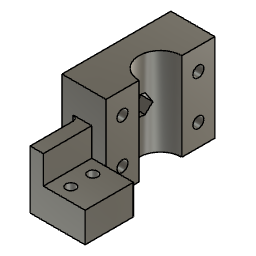
VI LC Clamp v1.0 (Autodesk Fusion 360 design; units mm, degrees)
Autodesk Fusion 360 part; units mm, degrees
note: some values were not read from the file. Set by a fixed rule: which sketch regions a step uses.
sketch "Sketch1" plane through (0, 0, 0) normal (0, 0, 1) x (1, 0, 0)
  circle A0 centre (0, 0) radius 9.75
  line L0 (0.0224, 9.75) -> (0.0224, 24.75)
  line L1 (0.0224, 24.75) -> (-19.9776, 24.75)
  line L2 (-19.9776, 24.75) -> (-19.9776, -24.75)
  line L3 (-19.9776, -24.75) -> (0, -24.75)
  line L4 (0, -24.75) -> (0, -9.75)
  line L5 (0, -24.75) -> (6.5, -24.75) construction
  line L6 (0, -24.75) -> (-6.5, -24.75) construction
  line L7 (-6.5, -24.75) -> (-6.5, -46.75)
  line L8 (-6.5, -46.75) -> (12.5, -46.75)
  line L9 (12.5, -46.75) -> (12.5, -25)
  line L10 (-6.5, -24.75) -> (-12.5, -24.75)
  line L11 (-12.5, -24.75) -> (-12.5, -46.75)
  line L12 (0, -24.75) -> (12.5, -24.75)
  line L13 (12.5, -24.75) -> (12.5, -25)
  line L14 (-6.5, -46.75) -> (-12.5, -46.75)
  dimension "d1" = 19.5
  dimension "d2" = 15
  dimension "d3" = 20
  dimension "d4" = 49.5
  dimension "d5" = 6.5
  dimension "d6" = 6.5
  dimension "d7" = 22
  dimension "d8" = 19
  dimension "d9" = 6
  constraint coincident A0.centre origin
  constraint coincident A0 L0.start
  constraint vertical L0
  constraint perpendicular L0 L1
  constraint perpendicular L1 L2
  constraint perpendicular L2 L3
  constraint coincident A0 L4.end
  constraint perpendicular L3 L4
  constraint perpendicular L4 L5
  constraint perpendicular L4 L6
  constraint perpendicular L3 L7
  constraint perpendicular L7 L8
  constraint perpendicular L8 L9
  constraint perpendicular L7 L10
  constraint perpendicular L3 L11
  constraint perpendicular L4 L12
  constraint perpendicular L11 L14
  measures "d1" diameter of A0
  measures "d2" distance of L0.start L0.end
  measures "d3" distance of L0.end L1.end
  measures "d4" distance of L1.end L2.end
  measures "d5" distance of L3.end L5.end
  measures "d6" distance of L3.end L6.end
  measures "d7" distance of L6.end L7.end
  measures "d8" distance of L7.end L8.end
  measures "d9" distance of L6.end L10.end
extrude "Extrude1" add sketch "Sketch1" along normal blind 40 contours A0 L0 L1 L2 L3 L4 L10
extrude "Extrude2" add sketch "Sketch1" along normal blind 13.6 contours L3 L7 L8 L9 L12 L13
extrude "Extrude3" add sketch "Sketch1" along normal blind 26.4 contours L3 L7 L10 L11 L14
sketch "Sketch2" plane through (-19.9776, 0, 0) normal (-1, 0, 0) x (0, -1, 0)
  line L0 (-24.75, 0) -> (24.75, 0)
  line L1 (24.75, 0) -> (24.75, 40)
  line L2 (24.75, 40) -> (-24.75, 40)
  line L3 (-24.75, 40) -> (-24.75, 0)
  line L4 (0, 40) -> (-9.75, 40) construction
  line L5 (-24.75, 40) -> (-17.25, 40) construction
  line L6 (-17.25, 40) -> (-17.25, 30) construction
  circle A0 centre (-17.25, 30) radius 2.5
  circle A1 centre (17.25, 30) radius 2.5
  circle A2 centre (-17.25, 10) radius 2.5
  circle A3 centre (17.25, 10) radius 2.5
  dimension "d16" = 9.75
  dimension "d17" = 7.5
  dimension "d18" = 10
  dimension "d20" = 5
  dimension "d23" = 34.5
  dimension "d24" = -20
  constraint midpoint L2 L4.start
  constraint perpendicular L1 L4
  constraint coincident L2.end L3.start
  constraint perpendicular L3 L5
  constraint perpendicular L0 L6
  constraint coincident L6.end A0.centre
  measures "d16" distance of L4.start L4.end
  measures "d17" distance of L2.end L5.end
  measures "d18" distance of L5.end L6.end
  measures "d20" diameter of A0
extrude "Extrude4" cut sketch "Sketch2" against normal blind 30 contours A0 | A1 | A2 | A3
sketch "Sketch3" plane through (0, 0, 13.6) normal (0, 0, 1) x (-1, 0, 0)
  line L0 (6.5, 24.75) -> (6.5, 46.75)
  line L1 (6.5, 46.75) -> (-12.5, 46.75)
  line L2 (-12.5, 46.75) -> (-12.5, 25)
  line L3 (0, 24.75) -> (6.5, 24.75)
  line L4 (-12.5, 25) -> (-12.5, 24.75)
  line L5 (-12.5, 24.75) -> (0, 24.75)
  line L6 (0, 24.75) -> (0, 30.75) construction
  circle A0 centre (0, 30.75) radius 2.25
  circle A1 centre (0, 40.75) radius 2.25
  dimension "d28" = 6
  dimension "d29" = 4.5
  dimension "d32" = 0
  dimension "d33" = 10
  constraint coincident L3.start L5.end
  constraint perpendicular L5 L6
  constraint coincident L6.end A0.centre
  measures "d28" distance of L3.start L6.end
  measures "d29" diameter of A0
extrude "Extrude5" cut sketch "Sketch3" against normal blind 14 contours A0 | A1
sketch "Sketch4" plane through (-19.9776, 0, 0) normal (-1, 0, 0) x (0, -1, 0)
  circle A0 centre (17.25, 30) radius 2.5
  circle A1 centre (17.25, 10) radius 2.5
  circle A2 centre (-17.25, 30) radius 2.5
  circle A3 centre (-17.25, 10) radius 2.5
  line L0 (-24.75, 0) -> (24.75, 0)
  line L1 (24.75, 0) -> (24.75, 40)
  line L2 (24.75, 40) -> (-24.75, 40)
  line L3 (-24.75, 40) -> (-24.75, 0)
  line L4 (0, 40) -> (0, 0) construction
  circle A4 centre (0, 20) radius 2.5
  dimension "d36" = 5
  constraint midpoint L2 L4.start
  constraint coincident L4.end origin
  constraint midpoint L4 A4.centre
  measures "d36" diameter of A4
extrude "Extrude6" cut sketch "Sketch4" against normal blind 20 contours A4
sketch "Sketch5" plane through (-19.9776, 0, 0) normal (-1, 0, 0) x (0, -1, 0)
  circle A0 centre (0, 20) radius 2.5
  circle A1 centre (17.25, 30) radius 2.5
  circle A2 centre (17.25, 10) radius 2.5
  circle A3 centre (-17.25, 30) radius 2.5
  circle A4 centre (-17.25, 10) radius 2.5
  line L0 (-24.75, 0) -> (24.75, 0)
  line L1 (24.75, 0) -> (24.75, 40)
  line L2 (24.75, 40) -> (-24.75, 40)
  line L3 (-24.75, 40) -> (-24.75, 0)
  line L4 (0, 20) -> (2.5, 24.3301) construction
  line L5 (0, 20) -> (5, 20) construction
  line L6 (0, 20) -> (-2.5, 24.3301) construction
  line L7 (0, 20) -> (5, 20) construction
  line L8 (0, 20) -> (-5, 20) construction
  line L9 (0, 20) -> (2.5, 15.6699) construction
  line L10 (-2.5, 15.6699) -> (0, 20) construction
  line L11 (5, 20) -> (2.5, 15.6699)
  line L12 (2.5, 15.6699) -> (-2.5, 15.6699)
  line L13 (-2.5, 15.6699) -> (-5, 20)
  line L14 (-5, 20) -> (-2.5, 24.3301)
  line L15 (-2.5, 24.3301) -> (2.5, 24.3301)
  line L16 (2.5, 24.3301) -> (5, 20)
  dimension "d40" = 60
  dimension "d41" = 5
  dimension "d42" = 120
  dimension "d43" = 5
  dimension "d44" = 5
  dimension "d45" = 5
  constraint coincident A0.centre L4.start
  constraint horizontal L5
  constraint horizontal L7
  constraint parallel L7 L8
  constraint parallel L6 L9
  constraint horizontal L12
  constraint parallel L11 L14
  constraint parallel L13 L16
  measures "d40" angle of L4 L5
  measures "d41" distance of A0.centre L4.end
  measures "d42" angle of L6 L7
  measures "d43" distance of A0.centre L6.end
  measures "d44" distance of A0.centre L8.end
  measures "d45" distance of A0.centre L9.end
extrude "Extrude7" cut sketch "Sketch5" against normal blind 7 from surface at -6 contours L11 L12 L13 L14 L15 L16
sketch "Sketch6" plane through (-19.9776, 0, 0) normal (-1, 0, 0) x (0, -1, 0)
  circle A0 centre (0, 20) radius 2.5
  circle A1 centre (17.25, 30) radius 2.5
  circle A2 centre (17.25, 10) radius 2.5
  circle A3 centre (-17.25, 30) radius 2.5
  circle A4 centre (-17.25, 10) radius 2.5
  line L0 (-24.75, 0) -> (24.75, 0)
  line L1 (24.75, 0) -> (24.75, 40)
  line L2 (24.75, 40) -> (-24.75, 40)
  line L3 (-24.75, 40) -> (-24.75, 0)
  circle A5 centre (-17.25, 30) radius 5
  circle A6 centre (17.25, 30) radius 5
  circle A7 centre (-17.25, 10) radius 5
  circle A8 centre (17.25, 10) radius 5
  dimension "d49" = 10
  dimension "d52" = 34.5
  dimension "d53" = -20
  constraint concentric A3 A5
  measures "d49" diameter of A5
extrude "Extrude8" cut sketch "Sketch6" against normal blind 3 contours A5 | A6 | A7 | A8
fillet "Fillet1" radius 2.5 1 edges at (-12.5, -24.75, 13.2)
